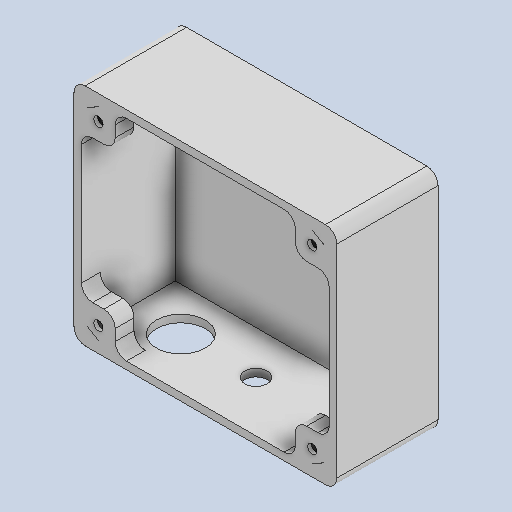
# Autodesk Inventor part: Kraicka_senzory
Saved by Autodesk Inventor 2025 (Build 290162000, 162)
## iProperties
Created: 2025-07-28
Part Number: Kraicka_senzory
Material: Generic
Document SubType Name: Modeling
Designer: Pravoslav
Density: 1 g/cm^3
Appearance: Default
Author: Pravoslav
Autodesk Inventor part; units mm, degrees
ref_plane "YZ Plane" through (0, 0, 0) normal (1, 0, 0) x (0, 1, 0)
ref_plane "XZ Plane" through (0, 0, 0) normal (0, 1, 0) x (-1, 0, 0)
ref_plane "XY Plane" through (0, 0, 0) normal (0, 0, 1) x (1, 0, 0)
sketch "Sketch1" plane through (0, 0, 0) normal (0, 0, 1) x (1, 0, 0)
  line L0 (-35, -30) -> (35, -30)
  line L1 (35, -30) -> (35, 30)
  line L2 (35, 30) -> (-35, 30)
  line L3 (-35, 30) -> (-35, -30)
  line L4 (-35, -30) -> (35, 30) construction
  line L5 (35, -30) -> (-35, 30) construction
  point P0 (0, 0)
  dimension "d0" = 70
  dimension "d1" = 60
  constraints: 12 end point, 2 midpoint, 2 parallel, 1 horizontal, 1 perpendicular
  measures "d0" distance of L2.end L1.end
  measures "d1" distance of L1.end L0.end
extrude "Extrusion1" add sketch "Sketch1" along normal blind 2
sketch "Sketch2" plane through (0, 0, 2) normal (0, 0, 1) x (1, 0, 0)
  line L0 (-35, -30) -> (35, -30) projected
  line L1 (-35, 30) -> (35, 30)
  line L2 (35, 30) -> (35, -30)
  line L3 (35, -30) -> (-35, -30)
  line L4 (-35, -30) -> (-35, 30)
  line L5 (-35, 30) -> (35, -30) construction
  line L6 (35, 30) -> (-35, -30) construction
  line L7 (-33, 28) -> (33, 28)
  line L8 (33, 28) -> (33, -28)
  line L9 (33, -28) -> (-33, -28)
  line L10 (-33, -28) -> (-33, 28)
  line L11 (-33, 28) -> (33, -28) construction
  line L12 (33, 28) -> (-33, -28) construction
  point P0 (0, 0)
  dimension "d4" = 2
  dimension "d5" = 2
  constraints: 24 end point, 4 midpoint, 4 parallel, 2 horizontal, 2 perpendicular
  measures "d4" distance between parallel lines of L0 L9
  measures "d5" distance between parallel lines of L2 L8
extrude "Extrusion2" add sketch "Sketch2" along normal blind 25
sketch "Sketch3" plane through (0, 0, 27) normal (0, 0, 1) x (1, 0, 0)
  line L0 (33, 28) -> (-33, 28) projected
  line L1 (-33, 28) -> (-24, 28)
  line L2 (-24, 28) -> (-24, 19)
  line L3 (-24, 19) -> (-33, 19)
  line L4 (-33, 19) -> (-33, 28)
  line L5 (33, 28) -> (33, -28) projected
  line L6 (33, 28) -> (24, 28)
  line L7 (24, 28) -> (24, 19)
  line L8 (24, 19) -> (33, 19)
  line L9 (33, 19) -> (33, 28)
  line L10 (-33, 28) -> (-33, -28) projected
  line L11 (-33, -28) -> (-24, -28)
  line L12 (-24, -28) -> (-24, -19)
  line L13 (-24, -19) -> (-33, -19)
  line L14 (-33, -19) -> (-33, -28)
  line L15 (33, -28) -> (24, -28)
  line L16 (24, -28) -> (24, -19)
  line L17 (24, -19) -> (33, -19)
  line L18 (33, -19) -> (33, -28)
  point P0 (0, 0)
  dimension "d8" = 9
  dimension "d9" = 9
  dimension "d10" = 9
  dimension "d11" = 9
  dimension "d12" = 9
  dimension "d13" = 9
  dimension "d14" = 9
  dimension "d15" = 9
  constraints: 32 end point, 8 parallel, 4 horizontal, 4 perpendicular, 2 point on line
  measures "d8" distance of L2.end L3.end
  measures "d9" distance of L1.end L2.end
  measures "d10" distance of L8.end L7.end
  measures "d11" distance of L7.end L6.end
  measures "d12" distance of L13.end L12.end
  measures "d13" distance of L12.end L11.end
  measures "d14" distance of L16.end L17.end
  measures "d15" distance of L15.end L16.end
extrude "Extrusion3" add sketch "Sketch3" against normal blind 5
sketch "Sketch4" plane through (0, 0, 27) normal (0, 0, 1) x (1, 0, 0)
  circle A0 centre (-28.5, 23.5) radius 3.45
  line L0 (-35, 30) -> (-35, -30) projected
  line L1 (35, 30) -> (-35, 30) projected
  line L2 (-31.4878, 21.775) -> (-31.4878, 25.225)
  line L3 (-31.4878, 25.225) -> (-28.5, 26.95)
  line L4 (-25.5122, 25.225) -> (-28.5, 26.95)
  line L5 (-25.5122, 25.225) -> (-25.5122, 21.775)
  line L6 (-25.5122, 21.775) -> (-28.5, 20.05)
  line L7 (-28.5, 20.05) -> (-31.4878, 21.775)
  point P0 (0, 0)
  dimension "d18" = 6.9
  dimension "d19" = 6.5
  dimension "d20" = 6.5
  dimension "d23" = 360
  constraints: 12 end point, 3 parallel, 1 vertical, 1 vertical alignment, 9 other
  measures "d19" distance from line of L0 point (-28.5, 23.5)
  measures "d20" distance from line of point (-28.5, 23.5) L1
extrude "Extrusion4" cut sketch "Sketch4" against normal blind 3.5 contours L5 L6 L7 L2 L3 L4
sketch "Sketch5" plane through (0, 0, 27) normal (0, 0, 1) x (1, 0, 0)
  line L0 (-28.5, 20.05) -> (-31.4878, 21.775) projected
  line L1 (-31.4878, 21.775) -> (-31.4878, 25.2078)
  line L2 (-28.5, 26.95) -> (-25.5122, 25.225) projected
  line L3 (-31.4878, 25.2078) -> (-28.5, 26.95)
  line L4 (-28.5, 26.95) -> (-25.5122, 25.225)
  line L5 (-25.5122, 25.225) -> (-25.5122, 21.775)
  line L6 (-25.5122, 21.775) -> (-28.4852, 20.0415)
  line L7 (-28.4852, 20.0415) -> (-31.4878, 21.775)
  circle A0 centre (-28.4852, 23.5085) radius 1.25
  point P0 (0, 0)
  dimension "d27" = 2.5
  constraints: 12 end point, 3 parallel, 1 centre point, 1 collinear, 1 vertical
  measures "d27" diameter of A0
extrude "Extrusion5" add sketch "Sketch5" against normal blind 1
mirror "Mirror1" about plane through (0, 0, 0) normal (1, 0, 0) of "Extrusion4"
mirror "Mirror2" about plane through (0, 0, 0) normal (1, 0, 0) of "Extrusion5"
mirror "Mirror3" about plane through (0, 0, 0) normal (0, 1, 0) of "Extrusion5", "Mirror2", "Extrusion4", "Mirror1"
sketch "Sketch6" plane through (-35, -30, 0) normal (0, -1, 0) x (1, 0, 0)
  circle A0 centre (15, 13.5) radius 6.5
  circle A1 centre (35, 13.5) radius 3
  line L0 (0, 27) -> (70, 27) projected
  line L1 (0, 0) -> (0, 27) projected
  point P0 (35, 0)
  dimension "d30" = 13
  dimension "d31" = 6
  dimension "d32" = 13.5
  dimension "d33" = 13.5
  dimension "d36" = 15
  dimension "d37" = 35
  constraints: 2 centre point
  measures "d30" diameter of A0
  measures "d31" diameter of A1
  measures "d32" distance from line of L0 A0.centre
  measures "d33" distance from line of A1.centre L0
  measures "d36" distance from line of L1 A0.centre
  measures "d37" distance from line of L1 A1.centre
extrude "Extrusion6" cut sketch "Sketch6" against normal up to surface (2 mm away)
fillet "Fillet1" radius 3 12 edges at (-33, -19, 24.5) (-24, -19, 24.5) (-24, -28, 24.5) (-33, 19, 24.5) (-24, 19, 24.5) (-24, 28, 24.5) (24, 28, 24.5) (24, 19, 24.5) (33, 19, 24.5) (33, -19, 24.5) (24, -19, 24.5) (24, -28, 24.5)
fillet "Fillet2" radius 3 4 edges at (-35, -30, 13.5) (35, -30, 13.5) (35, 30, 13.5) (-35, 30, 13.5)
body "Solid1"
